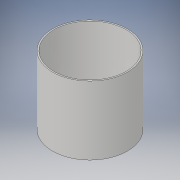
# Autodesk Inventor part: Base
Saved by Autodesk Inventor 2019 (Build 230136000, 136)
## iProperties
Created: 2020-02-03
Part Number: Base
Material: Generic
Document SubType Name: Modeling
Designer: Sergio
Density: 1 g/cm^3
Appearance: Default
Author: Sergio
Autodesk Inventor part; units mm, degrees
ref_plane "YZ Plane" through (0, 0, 0) normal (1, 0, 0) x (0, 1, 0)
ref_plane "XZ Plane" through (0, 0, 0) normal (0, 1, 0) x (-1, 0, 0)
ref_plane "XY Plane" through (0, 0, 0) normal (0, 0, 1) x (1, 0, 0)
sketch "Sketch1" plane through (0, 0, 0) normal (0, 1, 0) x (-1, 0, 0)
  circle A0 centre (0, 0) radius 49.1
  dimension "d12" = 98.2
  constraints: 1 centre point, 1 coincident
  measures "d12" diameter of A0
extrude "Extrusion1" add sketch "Sketch1" along normal blind 3
mirror "Mirror1" about plane through (0, 0, 0) normal (0, 0, 1)
sketch "Sketch10" plane through (0, 3, 0) normal (0, 1, 0) x (1, 0, 0)
  circle A0 centre (0, 0) radius 49.1
  circle A1 centre (0, 0) radius 50.9
  dimension "d23" = 101.8
  dimension "d52" = 1.8
  constraints: 2 centre point, 2 coincident
  measures "d23" diameter of A1
  measures "d52" radial gap between concentric circles of A0 A1
extrude "Extrusion4" add sketch "Sketch10" along normal blind 90 and the other way blind 3
sketch "Sketch13" plane through (0, 3, 0) normal (0, 1, 0) x (1, 0, 0)
  line L0 (-35, 13.5) -> (-26, 13.5)
  line L1 (-26, 13.5) -> (-26, 19.5)
  line L2 (-26, 19.5) -> (-35, 19.5)
  line L3 (-35, 19.5) -> (-35, 13.5)
  line L4 (-28, 14.5) -> (-33, 14.5)
  line L5 (-33, 14.5) -> (-33, 17.5)
  line L6 (-33, 17.5) -> (-28, 17.5)
  line L7 (-28, 17.5) -> (-28, 14.5)
  line L8 (0, 0) -> (0, 20.276) construction
  line L9 (-35, 13.5) -> (0, 13.5) construction
  dimension "d31" = 9
  dimension "d32" = 6
  dimension "d33" = 3
  dimension "d35" = 5
  dimension "d36" = 2
  dimension "d54" = 13.5
  dimension "d58" = 26
  constraints: 20 end point, 4 parallel, 3 perpendicular, 2 horizontal, 1 point on line, 1 vertical
  measures "d31" distance of L2.end L1.end
  measures "d32" distance of L1.end L0.end
  measures "d33" distance between parallel lines of L4 L6
  measures "d35" distance between parallel lines of L7 L5
  measures "d36" distance between parallel lines of L3 L5
  measures "d54" distance from line of L8.start L9
  measures "d58" distance between parallel lines of L8 L1
extrude "Extrusion6" add sketch "Sketch13" along normal blind 20
sketch "Sketch14" plane through (0, 3, 0) normal (0, 1, 0) x (1, 0, 0)
  line L0 (-33, 17.5) -> (-28, 17.5) projected
  line L1 (-28, 14.5) -> (-33, 14.5) projected
  line L2 (-33, 17.5) -> (-28, 17.5)
  line L3 (-28, 17.5) -> (-28, 14.5)
  line L4 (-28, 14.5) -> (-33, 14.5)
  line L5 (-33, 14.5) -> (-33, 17.5)
  point P0 (0, 0)
  constraints: 8 end point, 2 parallel, 1 horizontal, 1 perpendicular
extrude "Extrusion7" cut sketch "Sketch14" against normal blind 5
sketch "Sketch15" plane through (0, 23, 0) normal (0, 1, 0) x (1, 0, 0)
  line L0 (-35, 19.5) -> (-35, 13.5) projected
  line L1 (-35, 19.5) -> (-26, 19.5)
  line L2 (-26, 19.5) -> (-26, 13.5)
  line L3 (-26, 13.5) -> (-35, 13.5)
  line L4 (-35, 13.5) -> (-35, 19.5)
  point P0 (0, 0)
  constraints: 8 end point, 2 parallel, 1 horizontal, 1 perpendicular
extrude "Extrusion8" add sketch "Sketch15" along normal blind 2
sketch "Sketch17" plane through (0, 3, 0) normal (0, 1, 0) x (1, 0, 0)
  line L0 (48.6808, -6.9203) -> (46.2945, -6.9203)
  line L1 (46.2945, -6.9203) -> (46.2945, 6.9203)
  line L2 (46.2945, 6.9203) -> (48.6808, 6.9203)
  line L3 (48.6808, 6.9203) -> (48.6808, -6.9203)
  line L4 (48.6808, -6.9203) -> (46.2945, 6.9203) construction
  line L5 (46.2945, -6.9203) -> (48.6808, 6.9203) construction
  line L6 (44.5001, -13.602) -> (40.806, -13.602)
  line L7 (40.806, -13.602) -> (40.806, 13.602)
  line L8 (40.806, 13.602) -> (44.5001, 13.602)
  line L9 (44.5001, 13.602) -> (44.5001, -13.602)
  line L10 (44.5001, -13.602) -> (40.806, 13.602) construction
  line L11 (40.806, -13.602) -> (44.5001, 13.602) construction
  line L12 (38.6361, -9.1592) -> (35.6953, -9.1592)
  line L13 (35.6953, -9.1592) -> (35.6953, 9.1592)
  line L14 (35.6953, 9.1592) -> (38.6361, 9.1592)
  line L15 (38.6361, 9.1592) -> (38.6361, -9.1592)
  line L16 (38.6361, -9.1592) -> (35.6953, 9.1592) construction
  line L17 (35.6953, -9.1592) -> (38.6361, 9.1592) construction
  point P0 (0, 0)
  point P1 (47.4877, 0)
  point P2 (42.6531, 0)
  point P3 (37.1657, 0)
  constraints: 36 end point, 6 midpoint, 6 parallel, 3 horizontal, 3 perpendicular
extrude "Extrusion10" cut sketch "Sketch17" against normal blind 5
pattern_circular "Circular Pattern1" count 4 over 360 about axis through (0, -10, 0) along (0, 1, 0) of "Extrusion10"
sketch "Sketch18" plane through (0, 3, 0) normal (0, 1, 0) x (1, 0, 0)
  circle A0 centre (0, 0) radius 17.25
  dimension "d55" = 34.5
  constraints: 1 centre point, 1 coincident
  measures "d55" diameter of A0
extrude "Extrusion11" cut sketch "Sketch18" against normal blind 10
ref_plane "Work Plane1" through (0, 0, 0) normal (0, 0, 1) x (1, 0, 0)
body "Solid1"
